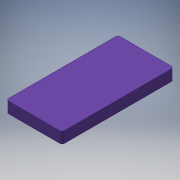
# Autodesk Inventor part: Piastra sostegno asse
Saved by Autodesk Inventor 2018 (Build 220112000, 112)
## iProperties
Created: 2020-06-01
Part Number: Piastra sostegno asse
Material: Generico
Document SubType Name: Modeling
Designer: Francesco
Density: 1 g/cm^3
Appearance: Violetto
Author: Francesco
Autodesk Inventor part; units mm, degrees
ref_plane "YZ Plane" through (0, 0, 0) normal (1, 0, 0) x (0, 1, 0)
ref_plane "XZ Plane" through (0, 0, 0) normal (0, 1, 0) x (-1, 0, 0)
ref_plane "XY Plane" through (0, 0, 0) normal (0, 0, 1) x (1, 0, 0)
sketch "Schizzo2" plane through (0, 0, 0) normal (0, 0, 1) x (1, 0, 0)
  line L0 (-25, 47.5) -> (25, 47.5)
  line L1 (25, 47.5) -> (25, -47.5)
  line L2 (25, -47.5) -> (-25, -47.5)
  line L3 (-25, -47.5) -> (-25, 47.5)
  line L4 (-25, 47.5) -> (25, -47.5) construction
  line L5 (25, 47.5) -> (-25, -47.5) construction
  point P0 (0, 0)
  dimension "d0" = 50
  dimension "d1" = 95
  constraints: 12 end point, 2 midpoint, 2 parallel, 1 horizontal, 1 perpendicular
  measures "d0" distance of L1.end L2.end
  measures "d1" distance of L0.end L1.end
extrude "Estrusione1" add sketch "Schizzo2" along normal blind 10
fillet "Raccordo1" radius 2 4 edges at (25, 47.5, 5) (-25, 47.5, 5) (25, -47.5, 5) (-25, -47.5, 5)
sketch "Schizzo3" plane through (0, 0, 0) normal (0, 0, -1) x (-1, 0, 0)
  line L0 (23, 47.5) -> (-23, 47.5) projected
  line L1 (25, -45.5) -> (25, 45.5) projected
  line L2 (-25, 45.5) -> (-25, -45.5) projected
  point P0 (0, 0)
  point P1 (15, 40.6)
  point P2 (-15, 40.6)
  dimension "d5" = 6.9
  dimension "d6" = 10
  dimension "d7" = 10
  constraints: 1 horizontal alignment
  measures "d5" distance from line of point (15, 40.6) L0
  measures "d6" distance from line of L1 point (15, 40.6)
  measures "d7" distance from line of L2 point (-15, 40.6)
hole "Foro1" at (-15, 40.6, 0) at (15, 40.6, 0) direction (0, 0, 1) diameter 5.5 end through all countersink diameter 10.4 countersink angle 90 clearance for "Vite a testa svasata piana ISO 2009/7046" size "M5" standard "ISO"
